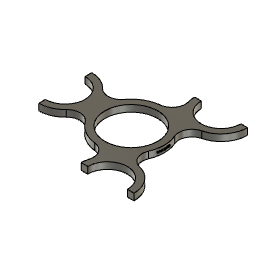
Model 25 (Autodesk Fusion 360 design; units mm, degrees)
Autodesk Fusion 360 part; units mm, degrees
sketch "Sketch1" plane through (0, 0, 0) normal (0, 0, 1) x (1, 0, 0)
  circle A0 centre (0, 0) radius 40
  line L0 (0, 0) -> (-100, 0) construction
  line L1 (0, 0) -> (50, 0) construction
  line L2 (50, 0) -> (50, 85.932) construction
  line L3 (50, 0) -> (50, -85.932) construction
  arc A1 (-71, 27.55) -> (-40.3571, 29.5178) centre (-56.5, 41.3249) ccw
  arc A2 (-5.519, 49.6945) -> (11.5156, 75.0255) centre (-7.7266, 69.5723) ccw
  arc A3 (59.5351, 47.0851) -> (45.9305, 19.7583) centre (64.3027, 27.6617) ccw
  arc A4 (45.9305, -19.7583) -> (59.5351, -47.0851) centre (64.3027, -27.6617) ccw
  arc A5 (11.5156, -75.0255) -> (-5.519, -49.6945) centre (-7.7266, -69.5723) ccw
  arc A6 (-40.3571, -29.5178) -> (-71, -27.55) centre (-56.5, -41.3249) ccw
  line L4 (-100, 0) -> (-100, 40) construction
  line L5 (-100, 0) -> (-100, -40) construction
  line L6 (50, 85.932) -> (90, 85.932) construction
  line L7 (50, 85.932) -> (10, 85.932) construction
  line L8 (50, -85.932) -> (90, -85.932) construction
  line L9 (50, -85.932) -> (10, -85.932) construction
  line L10 (20, -85.932) -> (10, -85.932)
  line L11 (80, -85.932) -> (90, -85.932)
  line L12 (-100, 30) -> (-100, 40)
  line L13 (-100, -30) -> (-100, -40)
  line L14 (20, 85.932) -> (10, 85.932)
  line L15 (90, 85.932) -> (80, 85.932)
  arc A7 (-100, -30) -> (-100, 30) centre (-100, 0) ccw
  arc A8 (20, 85.932) -> (80, 85.932) centre (50, 85.932) ccw
  arc A9 (80, -85.932) -> (20, -85.932) centre (50, -85.932) ccw
  arc A10 (-100, -40) -> (-71, -27.55) centre (-100, 0) ccw
  arc A11 (-71, 27.55) -> (-100, 40) centre (-100, 0) ccw
  arc A12 (10, 85.932) -> (11.5156, 75.0255) centre (50, 85.932) ccw
  arc A13 (59.5351, 47.0851) -> (90, 85.932) centre (50, 85.932) ccw
  arc A14 (90, -85.932) -> (59.5351, -47.0851) centre (50, -85.932) ccw
  arc A15 (11.5156, -75.0255) -> (10, -85.932) centre (50, -85.932) ccw
  arc A16 (-5.519, 49.6945) -> (-40.3571, 29.5178) centre (0, 0) ccw
  arc A17 (-40.3571, -29.5178) -> (-5.519, -49.6945) centre (0, 0) ccw
  arc A18 (45.9305, -19.7583) -> (45.9305, 19.7583) centre (0, 0) ccw
  dimension "d1" = 80
  dimension "d2" = 100
  dimension "d3" = 100
  dimension "d4" = 60
  dimension "d5" = 80
  dimension "d6" = 50
  dimension "d7" = 85.932
  dimension "d8" = 85.932
  dimension "d9" = 60
  dimension "d10" = 80
  dimension "d11" = 60
  dimension "d12" = 80
  dimension "d13" = 40
  dimension "d14" = 40
  dimension "d15" = 40
  dimension "d16" = 40
  dimension "d17" = 40
  dimension "d18" = 40
  constraint coincident A0.centre L0.start
  constraint horizontal L0
  constraint coincident L0.end L4.start
  constraint concentric A7 A10
  constraint parallel L0 L1
  constraint perpendicular L1 L2
  constraint perpendicular L1 L3
  constraint coincident L2.end L6.start
  constraint concentric A8 A12
  constraint coincident L3.end L8.start
  constraint concentric A9 A14
  constraint tangent A5 A17
  constraint tangent A5 A14
  constraint tangent A4 A17
  constraint tangent A4 A14
  constraint tangent A3 A12
  constraint tangent A3 A17
  constraint tangent A2 A17
  constraint tangent A2 A12
  constraint tangent A1 A10
  constraint tangent A1 A17
  constraint tangent A6 A10
  constraint tangent A6 A17
  constraint coincident A1.start A10
  constraint coincident A2.start A17
  constraint coincident A3.start A12
  constraint coincident A5.start A14
  constraint perpendicular L0 L4
  constraint perpendicular L0 L5
  constraint perpendicular L2 L6
  constraint parallel L6 L7
  constraint perpendicular L3 L8
  constraint parallel L8 L9
  constraint coincident L9 L10.start
  constraint coincident L8 L11.start
  constraint coincident L4 L12.start
  constraint coincident L5 L13.start
  constraint coincident L7 L14.start
  constraint coincident L6 L15.end
  constraint concentric A10 A11
  constraint concentric A12 A13
  constraint concentric A14 A15
  constraint concentric A16 A17
  constraint concentric A17 A18
  measures "d1" diameter of A0
  measures "d2" diameter of A17
  measures "d3" distance of A0.centre L0.end
  measures "d4" diameter of A7
  measures "d5" diameter of A10
  measures "d6" distance of A0.centre L1.end
  measures "d7" distance of L1.end L2.end
  measures "d8" distance of L1.end L3.end
  measures "d9" diameter of A8
  measures "d10" diameter of A12
  measures "d11" diameter of A9
  measures "d12" diameter of A14
  measures "d13" diameter of A1
  measures "d14" diameter of A2
  measures "d15" diameter of A3
  measures "d16" diameter of A4
  measures "d17" diameter of A5
  measures "d18" diameter of A6
extrude "Extrude1" add sketch "Sketch1" along normal blind 10
ref_plane "WorkPlane2" through (0, 0, 12.125) normal (1, 0, 0) x (0, 0, 1)
sketch "Sketch2" plane through (0, 0, 12.125) normal (1, 0, 0) x (0, 1, 0)
  line L0 (-15.9028, -10) -> (15, -10) construction
  line L1 (15, -10) -> (15, -3.5589) construction
  line L2 (15, -3.5589) -> (-15.9028, -3.5589) construction
  line L3 (-15.9028, -3.5589) -> (-15.9028, -10) construction
  text T0 "enes şahin" font "Arial" height 3 align centre middle in box 30.9028 x 6.4411 at (-15.9028, -10) x (1, 0) y (0, 1) spacing 1
extrude "Extrude2" add sketch "Sketch2" along normal blind 0.5 from the near side of the face at (49.7964, 4.5077, 6.6667) text T0
